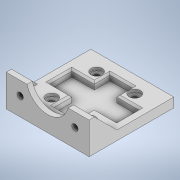
# Autodesk Inventor part: StepperMount
Saved by Autodesk Inventor 2020 (Build 240168000, 168)
## iProperties
Created: 2020-06-10
Part Number: StepperMount
Material: Generic
Document SubType Name: Modeling
Designer: Brandon
Density: 1 g/cm^3
Appearance: Default
Author: Brandon
Autodesk Inventor part; units mm, degrees
ref_plane "YZ Plane" through (0, 0, 0) normal (1, 0, 0) x (0, 1, 0)
ref_plane "XZ Plane" through (0, 0, 0) normal (0, 1, 0) x (-1, 0, 0)
ref_plane "XY Plane" through (0, 0, 0) normal (0, 0, 1) x (1, 0, 0)
sketch "Sketch1" plane through (0, 0, 0) normal (0, 0, 1) x (1, 0, 0)
  line L0 (0, 0) -> (47, 0)
  line L1 (47, 0) -> (47, 12.7)
  line L2 (47, 12.7) -> (0, 12.7)
  line L3 (0, 12.7) -> (0, 0)
  dimension "d0" = 47
  dimension "d1" = 12.7
  constraints: 8 end point, 2 parallel, 1 horizontal, 1 perpendicular
  measures "d0" distance of L1.end L2.end
  measures "d1" distance of L2.end L0.start
extrude "Extrusion1" add sketch "Sketch1" against normal blind 3
sketch "Sketch2" plane through (0, 0, 0) normal (0, -1, 0) x (1, 0, 0)
  line L0 (47, 0) -> (0, 0)
  line L1 (0, 0) -> (0, -48)
  line L2 (0, -48) -> (47, -48)
  line L3 (47, -48) -> (47, 0)
  line L4 (47, 0) -> (47, -3) projected
  line L5 (47, 0) -> (0, 0) projected
  dimension "d6" = 0
  dimension "d24" = 48
  dimension "d25" = 0
  constraints: 8 end point, 2 parallel, 1 horizontal, 1 perpendicular
  measures "d6" distance between parallel lines of L4 L3
  measures "d24" distance of L0.end L1.end
  measures "d25" distance between parallel lines of L0 L5
extrude "Extrusion2" add sketch "Sketch2" along normal blind 5.2832
sketch "Sketch3" plane through (0, 0, -3) normal (0, 0, -1) x (-1, 0, 0)
  line L0 (-47, 12.7) -> (-47, 0) projected
  line L1 (-47, 0) -> (0, 0) projected
  line L2 (-47, 12.7) -> (-45, 12.7)
  line L3 (-45, 12.7) -> (-45, 0)
  line L4 (-45, 0) -> (-47, 0)
  line L5 (-47, 0) -> (-47, 12.7)
  line L6 (0, 0) -> (0, 12.7) projected
  line L7 (0, 0) -> (-2, 0)
  line L8 (-2, 0) -> (-2, 12.7)
  line L9 (-2, 12.7) -> (0, 12.7)
  line L10 (0, 12.7) -> (0, 0)
  dimension "d7" = 2
  dimension "d8" = 2
  dimension "d9" = 12.7
  constraints: 16 end point, 4 parallel, 3 point on line, 2 horizontal, 2 perpendicular
  measures "d7" distance of L2.start L2.end
  measures "d8" distance of L8.end L9.end
  measures "d9" distance between parallel lines of L1 L2
extrude "Extrusion3" add sketch "Sketch3" along normal blind 12.7
chamfer "Chamfer1" distance 12.7 angle 45 2 edges at (46, 12.7, -15.7) (1, 12.7, -15.7)
sketch "Sketch4" plane through (0, 0, -3) normal (0, 0, -1) x (-1, 0, 0)
  circle A0 centre (-39.0056, 5.08) radius 1.75
  circle A1 centre (-8.0056, 5.08) radius 1.75
  line L0 (-45, 0) -> (-45, 12.7) projected
  line L1 (-2, 12.7) -> (-2, 0) projected
  line L2 (0, 0) -> (-47, 0) projected
  dimension "d15" = 3.5
  dimension "d16" = 3.5
  dimension "d17" = 5.9944
  dimension "d18" = 31
  dimension "d19" = 6.0056
  dimension "d20" = 5.08
  dimension "d21" = 5.08
  constraints: 2 centre point
  measures "d15" diameter of A0
  measures "d16" diameter of A1
  measures "d17" distance from line of L0 A0.centre
  measures "d18" distance of A1.centre A0.centre
  measures "d19" distance from line of L1 A1.centre
  measures "d20" distance from line of L2 A0.centre
  measures "d21" distance from line of L2 A1.centre
extrude "Extrusion4" cut sketch "Sketch4" against normal blind 12.7
sketch "Sketch5" plane through (0, 0, 0) normal (0, 0, 1) x (1, 0, 0)
  circle A0 centre (23.5, 15.7168) radius 12
  line L0 (47, -5.2832) -> (47, 12.7) projected
  line L1 (47, -5.2832) -> (0, -5.2832) projected
  point P0 (0, 0)
  dimension "d26" = 24
  dimension "d27" = 23.5
  dimension "d28" = 21
  constraints: 1 centre point
  measures "d26" diameter of A0
  measures "d27" distance from line of L0 A0.centre
  measures "d28" distance from line of L1 A0.centre
extrude "Extrusion5" cut sketch "Sketch5" against normal blind 5.2832
sketch "Sketch6" plane through (0, 0, 0) normal (0, 1, 0) x (1, 0, 0)
  circle A0 centre (12.7, 13.16) radius 1.5875
  circle A1 centre (12.7, 38.56) radius 1.5875
  circle A2 centre (34.3, 38.56) radius 1.5875
  circle A3 centre (34.3, 13.16) radius 1.5875
  line L0 (2, 3) -> (11.8854, 3) projected
  line L1 (0, 15.7) -> (0, 48) projected
  line L2 (47, 48) -> (47, 15.7) projected
  point P0 (0, 0)
  dimension "d31" = 3.175
  dimension "d32" = 3.175
  dimension "d33" = 3.175
  dimension "d34" = 3.175
  dimension "d35" = 10.16
  dimension "d36" = 25.4
  dimension "d37" = 25.4
  dimension "d38" = 10.16
  dimension "d39" = 12.7
  dimension "d40" = 12.7
  dimension "d41" = 12.7
  dimension "d42" = 12.7
  constraints: 4 centre point
  measures "d31" diameter of A0
  measures "d32" diameter of A1
  measures "d33" diameter of A3
  measures "d34" diameter of A2
  measures "d35" distance from line of L0 A0.centre
  measures "d36" distance of A0.centre A1.centre
  measures "d37" distance of A3.centre A2.centre
  measures "d38" distance from line of L0 A3.centre
  measures "d39" distance from line of L1 A0.centre
  measures "d40" distance from line of L1 A1.centre
  measures "d41" distance from line of L2 A3.centre
  measures "d42" distance from line of L2 A2.centre
extrude "Extrusion6" cut sketch "Sketch6" against normal blind 5.2832
sketch "Sketch7" plane through (0, 0, 0) normal (0, 1, 0) x (1, 0, 0)
  circle A0 centre (12.7, 13.16) radius 1.5875 projected
  circle A1 centre (12.7, 13.16) radius 3.175
  circle A2 centre (12.7, 38.56) radius 1.5875 projected
  circle A3 centre (12.7, 38.56) radius 3.175
  circle A4 centre (34.3, 13.16) radius 1.5875 projected
  circle A5 centre (34.3, 13.16) radius 3.175
  circle A6 centre (34.3, 38.56) radius 1.5875 projected
  circle A7 centre (34.3, 38.56) radius 3.175
  point P0 (0, 0)
  dimension "d45" = 6.35
  dimension "d46" = 6.35
  dimension "d47" = 6.35
  dimension "d48" = 6.35
  constraints: 4 centre point, 4 coincident
  measures "d45" diameter of A1
  measures "d46" diameter of A3
  measures "d47" diameter of A5
  measures "d48" diameter of A7
extrude "Extrusion7" cut sketch "Sketch7" against normal blind 1.4732 contours A0 | A1 | A2 | A3 | A4 | A5 | A6 | A7
chamfer "Chamfer2" distance 1.016 angle 45 4 edges at (11.1125, -1.4732, -13.16) (32.7125, -1.4732, -13.16) (11.1125, -1.4732, -38.56) (32.7125, -1.4732, -38.56)
sketch "Sketch8" plane through (0, 0, 0) normal (0, 1, 0) x (1, 0, 0)
  line L0 (4.445, 20.06) -> (42.545, 20.06)
  line L1 (42.545, 20.06) -> (42.545, 32.76)
  line L2 (42.545, 32.76) -> (4.445, 32.76)
  line L3 (4.445, 32.76) -> (4.445, 20.06)
  line L4 (17.145, 9.9) -> (29.845, 9.9)
  line L5 (29.845, 9.9) -> (29.845, 41.65)
  line L6 (29.845, 41.65) -> (17.145, 41.65)
  line L7 (17.145, 41.65) -> (17.145, 9.9)
  line L8 (0, 15.7) -> (0, 48) projected
  line L9 (47, 48) -> (47, 15.7) projected
  line L10 (0, 48) -> (47, 48) projected
  point P0 (0, 0)
  point P1 (17.145, 20.06)
  point P2 (29.845, 20.06)
  point P3 (29.845, 32.76)
  point P4 (17.145, 32.76)
  dimension "d54" = 12.7
  dimension "d55" = 38.1
  dimension "d56" = 4.445
  dimension "d57" = 4.455
  dimension "d58" = 15.24
  dimension "d59" = 12.7
  dimension "d60" = 17.145
  dimension "d61" = 17.155
  dimension "d62" = 31.75
  dimension "d63" = 6.35
  constraints: 16 end point, 4 parallel, 2 horizontal, 2 perpendicular
  measures "d54" distance of L2.end L0.start
  measures "d55" distance between parallel lines of L1 L3
  measures "d56" distance between parallel lines of L8 L3
  measures "d57" distance between parallel lines of L9 L1
  measures "d58" distance between parallel lines of L10 L2
  measures "d59" distance between parallel lines of L5 L7
  measures "d60" distance between parallel lines of L8 L7
  measures "d61" distance between parallel lines of L9 L5
  measures "d62" distance between parallel lines of L6 L4
  measures "d63" distance between parallel lines of L10 L6
extrude "Extrusion8" cut sketch "Sketch8" against normal blind 3.81
chamfer "Chamfer3" distance 1.016 angle 45 12 edges at (10.795, 0, -20.06) (4.445, 0, -26.41) (10.795, 0, -32.76) (17.145, 0, -37.205) (23.495, 0, -41.65) (29.845, 0, -37.205) (36.195, 0, -32.76) (42.545, 0, -26.41) (36.195, 0, -20.06) (29.845, 0, -14.98) (23.495, 0, -9.9) (17.145, 0, -14.98)
body "Solid1"
